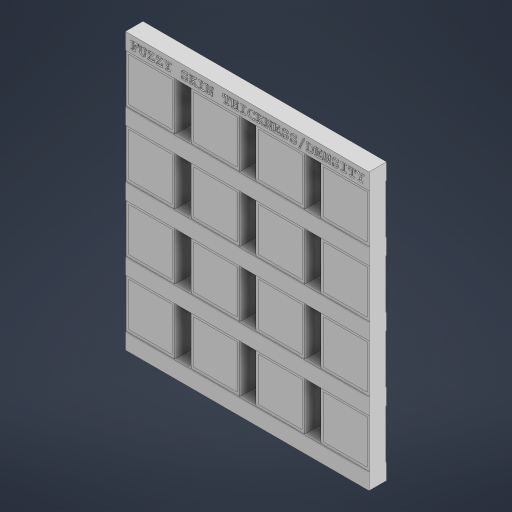
# Autodesk Inventor part: Fuzzy Skin Swatch Module
Saved by Autodesk Inventor 2023.1 (Build 271208000, 208)
## iProperties
Created: 2022-11-27
Part Number: Fuzzy Skin Swatch Module
Material: Generic
Document SubType Name: Modeling
Designer: aubrey-work
Density: 1 g/cm^3
Appearance: Default
Author: aubrey-work
Autodesk Inventor part; units mm, degrees
(part 1 of 2)
ref_plane "YZ Plane" through (0, 0, 0) normal (1, 0, 0) x (0, 1, 0)
ref_plane "XZ Plane" through (0, 0, 0) normal (0, 1, 0) x (-1, 0, 0)
sketch "Sketch1" plane through (0, 0, 0) normal (0, 1, 0) x (-1, 0, 0)
  line L0 (10, -2.7) -> (-10, -2.7)
  line L1 (-10, -2.7) -> (-10, 2.7)
  line L2 (-10, 2.7) -> (10, 2.7)
  line L3 (10, 2.7) -> (10, -2.7)
  line L4 (10, -2.7) -> (-10, 2.7) construction
  line L5 (-10, -2.7) -> (10, 2.7) construction
  point P0 (0, 0)
  dimension "d0" = 20
  dimension "d1" = 5.4
  constraints: 12 end point, 2 midpoint, 2 parallel, 1 horizontal, 1 perpendicular
  measures "d0" distance of L1.end L2.end
  measures "d1" distance of L0.end L1.end
extrude "Bottom Label" add sketch "Sketch1" along normal blind 5
sketch "Sketch2" plane through (0, 5, 0) normal (0, 1, 0) x (1, 0, 0)
  line L0 (-10, -2.5) -> (5, -2.5)
  line L1 (5, -2.5) -> (5, 2.5)
  line L2 (5, 2.5) -> (-10, 2.5)
  line L3 (-10, 2.5) -> (-10, -2.5)
  line L4 (-10, -2.5) -> (5, 2.5) construction
  line L5 (5, -2.5) -> (-10, 2.5) construction
  line L6 (-10, 2.7) -> (-10, -2.7) projected
  point P0 (-2.5, 0)
  point P1 (-2.5, 0)
  point P2 (-10, 0)
  dimension "d4" = 15
  dimension "d5" = 5
  constraints: 12 end point, 4 midpoint, 2 parallel, 1 coincident, 1 horizontal, 1 perpendicular
  measures "d4" distance of L2.end L1.end
  measures "d5" distance of L1.end L0.end
extrude "Tile" add sketch "Sketch2" along normal blind 15
sketch "Sketch7" plane through (-10, 5, 2.5) normal (0, 0, 1) x (1, 0, 0)
  line L0 (15, 0) -> (0, 0) projected
  line L1 (15, 0) -> (15, 15) projected
  line L2 (0, 15) -> (15, 15) projected
  line L3 (0, 0) -> (0, 15) projected
  line L4 (14.2, 14.2) -> (14.2, 0.8)
  line L5 (14.2, 0.8) -> (0.8, 0.8)
  line L6 (0.8, 0.8) -> (0.8, 14.2)
  line L7 (0.8, 14.2) -> (14.2, 14.2)
  point P0 (10, -5)
  dimension "d28" = 0.8
  constraints: 8 end point, 3 other
  measures "d28" distance between parallel lines of L2 L7
extrude "Cut Tile" cut sketch "Sketch7" against normal blind 4.2 contours L4 L5 L6 L7
extrude "Create Tile Inset" add sketch "Sketch7" against normal blind 4.2 separate body contours L4 L5 L6 L7
pattern_linear "Frame Pattern" count 4 spacing 20 along (1, 0, 0) count 4 spacing 20 along (0, 1, 0) of "Tile", "Bottom Label", "Cut Tile" bodies 1
pattern_linear "Tile Insets Rectangular Pattern" count 4 spacing 20 along (1, 0, 0) count 4 spacing 20 along (0, 1, 0) of "Create Tile Inset" bodies 2
sketch "Sketch5" plane through (0, 0, 0) normal (0, 1, 0) x (-1, 0, 0)
  line L0 (-65, 2.7) -> (-70, 2.7)
  line L1 (-70, 2.7) -> (-70, -2.7)
  line L2 (-70, -2.7) -> (-65, -2.7)
  line L3 (-65, -2.7) -> (-65, 2.7)
  line L4 (-65, 2.7) -> (-70, -2.7) construction
  line L5 (-70, 2.7) -> (-65, -2.7) construction
  line L6 (10, -2.7) -> (10, 2.7) projected
  line L7 (6.3576, 0) -> (13.6424, 0) construction
  line L8 (-65, 0) -> (-70, 0) construction
  point P0 (0, 0)
  point P1 (-67.5, 0)
  point P2 (10, 0)
  dimension "d21" = 5
  dimension "d22" = 5.4
  dimension "d23" = 80
  constraints: 16 end point, 6 midpoint, 2 horizontal, 2 parallel, 1 collinear, 1 perpendicular
  measures "d21" distance of L2.end L1.end
  measures "d22" distance of L1.end L0.end
  measures "d23" distance between parallel lines of L6 L1
extrude "Trim Portruding Labels" cut sketch "Sketch5" along normal through all bodies 1
ref_plane "Work Plane1" through (0, 80, 0) normal (0, -1, 0) x (1, 0, 0)
sketch "Sketch6" plane through (0, 80, 0) normal (0, -1, 0) x (1, 0, 0)
  line L0 (65, -2.7) -> (65, 2.7) projected
  line L1 (-10, 2.7) -> (65, 2.7) projected
  line L2 (-10, -2.7) -> (-10, 2.7) projected
  line L3 (65, -2.7) -> (-10, -2.7) projected
  point P0 (0, 0)
extrude "Top Label" add sketch "Sketch6" against normal blind 5 bodies 1
sketch "Sketch4" plane through (-10, 80, 2.7) normal (0, 0, 1) x (1, 0, 0)
  line L0 (0, 5) -> (75, 5) projected
  line L1 (75, 5) -> (75, 0) projected
  line L2 (75, 0) -> (0, 0) projected
  line L3 (0, 0) -> (0, 5) projected
  line L4 (75, -20) -> (0, -20) projected
  line L5 (0, -20) -> (0, -15) projected
  line L6 (0, -15) -> (75, -15) projected
  line L7 (75, -40) -> (0, -40) projected
  line L8 (0, -40) -> (0, -35) projected
  line L9 (0, -35) -> (75, -35) projected
  line L10 (75, -60) -> (0, -60) projected
  line L11 (0, -60) -> (0, -55) projected
  line L12 (0, -55) -> (75, -55) projected
  line L13 (75, -80) -> (0, -80) projected
  line L14 (0, -80) -> (0, -75) projected
  line L15 (0, -75) -> (75, -75) projected
  line L16 (75, -15) -> (75, -20) projected
  line L17 (75, -35) -> (75, -40) projected
  line L18 (75, -55) -> (75, -60) projected
  line L19 (75, -75) -> (75, -80) projected
  line L20 (2.4665, 2.0577) -> (2.4665, 1.4293)
  line L21 (2.4665, 1.4293) -> (2.9052, 1.4293)
  spline S0 degree 2 poles (2.9052, 1.4293) (3.0665, 1.4293) (3.1993, 1.3107) (3.1993, 1.2134) knots 0 0 0 1 2 2 2
  spline S1 degree 2 poles (3.1993, 1.2134) (3.1993, 1.1162) (3.0665, 1) (2.9052, 1) knots 0 0 0 1 2 2 2
  line L22 (2.9052, 1) -> (1.9708, 1)
  spline S2 degree 2 poles (1.9708, 1) (1.8096, 1) (1.6767, 1.1186) (1.6767, 1.2158) knots 0 0 0 1 2 2 2
  spline S3 degree 2 poles (1.6767, 1.2158) (1.6767, 1.3131) (1.8096, 1.4293) (1.9708, 1.4293) knots 0 0 0 1 2 2 2
  line L23 (1.9708, 1.4293) -> (2.0372, 1.4293)
  line L24 (2.0372, 1.4293) -> (2.0372, 3.1107)
  line L25 (2.0372, 3.1107) -> (1.9708, 3.1107)
  spline S4 degree 2 poles (1.9708, 3.1107) (1.8096, 3.1107) (1.6767, 3.2293) (1.6767, 3.3266) knots 0 0 0 1 2 2 2
  spline S5 degree 2 poles (1.6767, 3.3266) (1.6767, 3.4214) (1.8096, 3.54) (1.9708, 3.54) knots 0 0 0 1 2 2 2
  line L26 (1.9708, 3.54) -> (3.9914, 3.5376)
  line L27 (3.9914, 3.5376) -> (3.9914, 2.8854)
  spline S6 degree 2 poles (3.9914, 2.8854) (3.9914, 2.7242) (3.8729, 2.5914) (3.7756, 2.5914) knots 0 0 0 1 2 2 2
  spline S7 degree 2 poles (3.7756, 2.5914) (3.6784, 2.5914) (3.5622, 2.7242) (3.5622, 2.8854) knots 0 0 0 1 2 2 2
  line L28 (3.5622, 2.8854) -> (3.5622, 3.1107)
  line L29 (3.5622, 3.1107) -> (2.4665, 3.1107)
  line L30 (2.4665, 3.1107) -> (2.4665, 2.487)
  line L31 (2.4665, 2.487) -> (2.8436, 2.487)
  spline S8 degree 2 poles (2.8436, 2.487) (2.8436, 2.6483) (2.8815, 2.691) knots 0 0 0 1 1 1
  spline S9 degree 2 poles (2.8815, 2.691) (2.9622, 2.7811) (3.0594, 2.7811) knots 0 0 0 1 1 1
  spline S10 degree 2 poles (3.0594, 2.7811) (3.1566, 2.7811) (3.2728, 2.6483) (3.2728, 2.487) knots 0 0 0 1 2 2 2
  line L32 (3.2728, 2.487) -> (3.2728, 2.0577)
  spline S11 degree 2 poles (3.2728, 2.0577) (3.2728, 1.8965) (3.1543, 1.7637) (3.057, 1.7637) knots 0 0 0 1 2 2 2
  spline S12 degree 2 poles (3.057, 1.7637) (2.9598, 1.7637) (2.8815, 1.8538) knots 0 0 0 1 1 1
  spline S13 degree 2 poles (2.8815, 1.8538) (2.8436, 1.8965) (2.8436, 2.0577) knots 0 0 0 1 1 1
  line L33 (2.8436, 2.0577) -> (2.4665, 2.0577)
  line L34 (6.3156, 3.1084) -> (6.3156, 1.8917)
  spline S14 degree 2 poles (6.3156, 1.8917) (6.3156, 1.4957) (5.7441, 0.9383) (5.3433, 0.9383) knots 0 0 0 1 2 2 2
  spline S15 degree 2 poles (5.3433, 0.9383) (5.1441, 0.9383) (4.7954, 1.0783) (4.5156, 1.351) (4.3614, 1.6451) (4.3614, 1.8917) knots 0 0 0 1 2 3 4 4 4
  line L35 (4.3614, 1.8917) -> (4.3614, 3.1084)
  spline S16 degree 2 poles (4.3614, 3.1084) (4.2001, 3.1084) (4.0673, 3.2269) (4.0673, 3.3242) knots 0 0 0 1 2 2 2
  spline S17 degree 2 poles (4.0673, 3.3242) (4.0673, 3.4214) (4.2001, 3.5376) (4.3614, 3.5376) knots 0 0 0 1 2 2 2
  line L36 (4.3614, 3.5376) -> (4.9448, 3.54)
  spline S18 degree 2 poles (4.9448, 3.54) (5.0848, 3.54) (5.2176, 3.4214) (5.2176, 3.3266) knots 0 0 0 1 2 2 2
  spline S19 degree 2 poles (5.2176, 3.3266) (5.2176, 3.2293) (5.0848, 3.1107) (4.9448, 3.1107) knots 0 0 0 1 2 2 2
  line L37 (4.9448, 3.1107) -> (4.7907, 3.1107)
  line L38 (4.7907, 3.1107) -> (4.7907, 1.8562)
  spline S20 degree 2 poles (4.7907, 1.8562) (4.7907, 1.6641) (5.1108, 1.3676) (5.3362, 1.3676) knots 0 0 0 1 2 2 2
  spline S21 degree 2 poles (5.3362, 1.3676) (5.4879, 1.3676) (5.7512, 1.5099) (5.8342, 1.6475) knots 0 0 0 1 2 2 2
  spline S22 degree 2 poles (5.8342, 1.6475) (5.8864, 1.7328) (5.8864, 1.8562) knots 0 0 0 1 1 1
  line L39 (5.8864, 1.8562) -> (5.8864, 3.1107)
  line L40 (5.8864, 3.1107) -> (5.7322, 3.1107)
  spline S23 degree 2 poles (5.7322, 3.1107) (5.5923, 3.1107) (5.4595, 3.2293) (5.4595, 3.3266) knots 0 0 0 1 2 2 2
  spline S24 degree 2 poles (5.4595, 3.3266) (5.4595, 3.4214) (5.5923, 3.54) (5.7322, 3.54) knots 0 0 0 1 2 2 2
  line L41 (5.7322, 3.54) -> (6.3156, 3.5376)
  spline S25 degree 2 poles (6.3156, 3.5376) (6.4769, 3.5376) (6.6097, 3.4214) (6.6097, 3.3242) knots 0 0 0 1 2 2 2
  spline S26 degree 2 poles (6.6097, 3.3242) (6.6097, 3.2269) (6.4769, 3.1084) (6.3156, 3.1084) knots 0 0 0 1 2 2 2
  line L42 (7.4848, 1.4293) -> (8.4596, 1.4293)
  line L43 (8.4596, 1.4293) -> (8.4596, 1.7471)
  spline S27 degree 2 poles (8.4596, 1.7471) (8.4596, 1.9083) (8.5782, 2.0411) (8.6754, 2.0411) knots 0 0 0 1 2 2 2
  spline S28 degree 2 poles (8.6754, 2.0411) (8.7703, 2.0411) (8.8888, 1.9083) (8.8888, 1.7471) knots 0 0 0 1 2 2 2
  line L44 (8.8888, 1.7471) -> (8.8865, 1)
  line L45 (8.8865, 1) -> (6.937, 1)
  line L46 (6.937, 1) -> (6.937, 1.4293)
  line L47 (6.937, 1.4293) -> (8.2438, 3.1107)
  line L48 (8.2438, 3.1107) -> (7.4564, 3.1107)
  line L49 (7.4564, 3.1107) -> (7.4564, 2.8024)
  spline S29 degree 2 poles (7.4564, 2.8024) (7.4564, 2.6412) (7.3402, 2.5083) (7.2429, 2.5083) knots 0 0 0 1 2 2 2
  spline S30 degree 2 poles (7.2429, 2.5083) (7.1457, 2.5083) (7.0271, 2.6412) (7.0271, 2.8024) knots 0 0 0 1 2 2 2
  line L50 (7.0271, 2.8024) -> (7.0271, 3.54)
  line L51 (7.0271, 3.54) -> (8.7987, 3.5376)
  line L52 (8.7987, 3.5376) -> (8.7987, 3.1202)
  line L53 (8.7987, 3.1202) -> (7.4848, 1.4293)
  line L54 (10.058, 1.4293) -> (11.0328, 1.4293)
  line L55 (11.0328, 1.4293) -> (11.0328, 1.7471)
  spline S31 degree 2 poles (11.0328, 1.7471) (11.0328, 1.9083) (11.1514, 2.0411) (11.2486, 2.0411) knots 0 0 0 1 2 2 2
  spline S32 degree 2 poles (11.2486, 2.0411) (11.3435, 2.0411) (11.462, 1.9083) (11.462, 1.7471) knots 0 0 0 1 2 2 2
  line L56 (11.462, 1.7471) -> (11.4597, 1)
  line L57 (11.4597, 1) -> (9.5102, 1)
  line L58 (9.5102, 1) -> (9.5102, 1.4293)
  line L59 (9.5102, 1.4293) -> (10.817, 3.1107)
  line L60 (10.817, 3.1107) -> (10.0296, 3.1107)
  line L61 (10.0296, 3.1107) -> (10.0296, 2.8024)
  spline S33 degree 2 poles (10.0296, 2.8024) (10.0296, 2.6412) (9.9134, 2.5083) (9.8161, 2.5083) knots 0 0 0 1 2 2 2
  spline S34 degree 2 poles (9.8161, 2.5083) (9.7189, 2.5083) (9.6003, 2.6412) (9.6003, 2.8024) knots 0 0 0 1 2 2 2
  line L62 (9.6003, 2.8024) -> (9.6003, 3.54)
  line L63 (9.6003, 3.54) -> (11.3719, 3.5376)
  line L64 (11.3719, 3.5376) -> (11.3719, 3.1202)
  line L65 (11.3719, 3.1202) -> (10.058, 1.4293)
  line L66 (13.2716, 2.0649) -> (13.2716, 1.4293)
  line L67 (13.2716, 1.4293) -> (13.5609, 1.4293)
  spline S35 degree 2 poles (13.5609, 1.4293) (13.7222, 1.4293) (13.855, 1.3107) (13.855, 1.2134) knots 0 0 0 1 2 2 2
  spline S36 degree 2 poles (13.855, 1.2134) (13.855, 1.1162) (13.7222, 1) (13.5609, 1) knots 0 0 0 1 2 2 2
  line L68 (13.5609, 1) -> (12.553, 1)
  spline S37 degree 2 poles (12.553, 1) (12.3917, 1) (12.2589, 1.1186) (12.2589, 1.2158) knots 0 0 0 1 2 2 2
  spline S38 degree 2 poles (12.2589, 1.2158) (12.2589, 1.3131) (12.3917, 1.4293) (12.553, 1.4293) knots 0 0 0 1 2 2 2
  line L69 (12.553, 1.4293) -> (12.8423, 1.4293)
  line L70 (12.8423, 1.4293) -> (12.8423, 2.0649)
  line L71 (12.8423, 2.0649) -> (12.1308, 3.1131)
  spline S39 degree 2 poles (12.1308, 3.1131) (11.9696, 3.1131) (11.8368, 3.2317) (11.8368, 3.3289) knots 0 0 0 1 2 2 2
  spline S40 degree 2 poles (11.8368, 3.3289) (11.8368, 3.4238) (11.9696, 3.5424) (12.1308, 3.5424) knots 0 0 0 1 2 2 2
  line L72 (12.1308, 3.5424) -> (12.534, 3.54)
  spline S41 degree 2 poles (12.534, 3.54) (12.6905, 3.54) (12.8233, 3.4238) (12.8233, 3.3266) knots 0 0 0 1 2 2 2
  spline S42 degree 2 poles (12.8233, 3.3266) (12.8233, 3.1819) (12.6502, 3.1107) knots 0 0 0 1 1 1
  line L73 (12.6502, 3.1107) -> (13.0581, 2.5107)
  line L74 (13.0581, 2.5107) -> (13.4637, 3.1107)
  spline S43 degree 2 poles (13.4637, 3.1107) (13.3024, 3.1107) (13.1696, 3.2293) (13.1696, 3.3266) knots 0 0 0 1 2 2 2
  spline S44 degree 2 poles (13.1696, 3.3266) (13.1696, 3.4214) (13.3024, 3.54) (13.4637, 3.54) knots 0 0 0 1 2 2 2
  line L75 (13.4637, 3.54) -> (13.9807, 3.54)
  spline S45 degree 2 poles (13.9807, 3.54) (14.1396, 3.54) (14.2724, 3.4238) (14.2724, 3.3266) knots 0 0 0 1 2 2 2
  spline S46 degree 2 poles (14.2724, 3.3266) (14.2724, 3.2293) (14.1396, 3.1107) (13.9807, 3.1107) knots 0 0 0 1 2 2 2
  line L76 (13.9807, 3.1107) -> (13.2716, 2.0649)
  spline S47 degree 2 poles (17.5737, 1.1091) (17.5168, 1.0427) (17.448, 1.0047) (17.3982, 1.0047) knots 0 0 0 1 2 2 2
  spline S48 degree 2 poles (17.3982, 1.0047) (17.2986, 1.0047) (17.18, 1.1376) (17.18, 1.2893) knots 0 0 0 1 2 2 2
  line L77 (17.18, 1.2893) -> (17.18, 1.5787)
  spline S49 degree 2 poles (17.18, 1.5787) (17.18, 1.7328) (17.2986, 1.8656) (17.3982, 1.8656) knots 0 0 0 1 2 2 2
  spline S50 degree 2 poles (17.3982, 1.8656) (17.4741, 1.8656) (17.5761, 1.785) (17.6306, 1.6) (17.6591, 1.5668) knots 0 0 0 1 2 3 3 3
  spline S51 degree 2 poles (17.6591, 1.5668) (17.7207, 1.5004) (18.029, 1.3676) (18.2117, 1.3676) knots 0 0 0 1 2 2 2
  spline S52 degree 2 poles (18.2117, 1.3676) (18.4986, 1.3676) (18.6836, 1.5004) knots 0 0 0 1 1 1
  spline S53 degree 2 poles (18.6836, 1.5004) (18.7998, 1.5834) (18.7998, 1.702) knots 0 0 0 1 1 1
  spline S54 degree 2 poles (18.7998, 1.702) (18.7998, 1.7826) (18.6883, 1.9226) (18.5603, 1.9676) knots 0 0 0 1 2 2 2
  spline S55 degree 2 poles (18.5603, 1.9676) (18.4773, 1.9985) (18.1879, 2.053) knots 0 0 0 1 1 1
  spline S56 degree 2 poles (18.1879, 2.053) (17.8369, 2.1194) (17.4765, 2.302) (17.2654, 2.6364) (17.2654, 2.8309) knots 0 0 0 1 2 3 3 3
  spline S57 degree 2 poles (17.2654, 2.8309) (17.2654, 3.1392) (17.78, 3.6017) (18.1927, 3.6017) knots 0 0 0 1 2 2 2
  spline S58 degree 2 poles (18.1927, 3.6017) (18.3587, 3.6017) (18.6409, 3.5281) (18.7571, 3.4523) knots 0 0 0 1 2 2 2
  spline S59 degree 2 poles (18.7571, 3.4523) (18.8401, 3.5353) (18.9255, 3.5353) knots 0 0 0 1 1 1
  spline S60 degree 2 poles (18.9255, 3.5353) (19.0204, 3.5353) (19.139, 3.4024) (19.139, 3.2507) knots 0 0 0 1 2 2 2
  line L78 (19.139, 3.2507) -> (19.139, 2.9281)
  spline S61 degree 2 poles (19.139, 2.9281) (19.139, 2.774) (19.0204, 2.6412) (18.9255, 2.6412) knots 0 0 0 1 2 2 2
  spline S62 degree 2 poles (18.9255, 2.6412) (18.8472, 2.6412) (18.788, 2.6886) knots 0 0 0 1 1 1
  spline S63 degree 2 poles (18.788, 2.6886) (18.7405, 2.7242) (18.6955, 2.9376) (18.6599, 2.985) knots 0 0 0 1 2 2 2
  spline S64 degree 2 poles (18.6599, 2.985) (18.5982, 3.0633) (18.3563, 3.1724) (18.1974, 3.1724) knots 0 0 0 1 2 2 2
  spline S65 degree 2 poles (18.1974, 3.1724) (17.965, 3.1724) (17.6946, 2.9566) (17.6946, 2.8404) knots 0 0 0 1 2 2 2
  spline S66 degree 2 poles (17.6946, 2.8404) (17.6946, 2.7597) (17.8061, 2.6127) (17.9105, 2.57) knots 0 0 0 1 2 2 2
  spline S67 degree 2 poles (17.9105, 2.57) (17.9816, 2.5416) (18.6385, 2.4111) (18.9943, 2.257) (19.2291, 1.9249) (19.2291, 1.6973) knots 0 0 0 1 2 3 4 4 4
  spline S68 degree 2 poles (19.2291, 1.6973) (19.2291, 1.3795) (19.0061, 1.1897) knots 0 0 0 1 1 1
  spline S69 degree 2 poles (19.0061, 1.1897) (18.7073, 0.9383) (18.2472, 0.9383) knots 0 0 0 1 1 1
  spline S70 degree 2 poles (18.2472, 0.9383) (18.0694, 0.9383) (17.7326, 1.0237) (17.5737, 1.1091) knots 0 0 0 1 2 2 2
  line L79 (20.3271, 1.9083) -> (20.3271, 1.4293)
  line L80 (20.3271, 1.4293) -> (20.4813, 1.4293)
  spline S71 degree 2 poles (20.4813, 1.4293) (20.6212, 1.4293) (20.754, 1.3107) (20.754, 1.2134) knots 0 0 0 1 2 2 2
  spline S72 degree 2 poles (20.754, 1.2134) (20.754, 1.1162) (20.6212, 1) (20.4813, 1) knots 0 0 0 1 2 2 2
  line L81 (20.4813, 1) -> (19.8315, 1)
  spline S73 degree 2 poles (19.8315, 1) (19.6915, 1) (19.5587, 1.1186) (19.5587, 1.2158) knots 0 0 0 1 2 2 2
  spline S74 degree 2 poles (19.5587, 1.2158) (19.5587, 1.3131) (19.6915, 1.4293) (19.8315, 1.4293) knots 0 0 0 1 2 2 2
  line L82 (19.8315, 1.4293) -> (19.8979, 1.4293)
  line L83 (19.8979, 1.4293) -> (19.8979, 3.1107)
  line L84 (19.8979, 3.1107) -> (19.8315, 3.1107)
  spline S75 degree 2 poles (19.8315, 3.1107) (19.6915, 3.1107) (19.5587, 3.2293) (19.5587, 3.3266) knots 0 0 0 1 2 2 2
  spline S76 degree 2 poles (19.5587, 3.3266) (19.5587, 3.4214) (19.6915, 3.54) (19.8315, 3.54) knots 0 0 0 1 2 2 2
  line L85 (19.8315, 3.54) -> (20.4813, 3.5376)
  spline S77 degree 2 poles (20.4813, 3.5376) (20.6212, 3.5376) (20.754, 3.4214) (20.754, 3.3242) knots 0 0 0 1 2 2 2
  spline S78 degree 2 poles (20.754, 3.3242) (20.754, 3.2269) (20.6212, 3.1084) (20.4813, 3.1084) knots 0 0 0 1 2 2 2
  line L86 (20.4813, 3.1084) -> (20.3271, 3.1084)
  line L87 (20.3271, 3.1084) -> (20.3271, 2.4728)
  line L88 (20.3271, 2.4728) -> (21.0884, 3.1273)
  spline S79 degree 2 poles (21.0884, 3.1273) (21.1027, 3.1273) (20.9698, 3.2246) (20.9698, 3.3218) knots 0 0 0 1 2 2 2
  spline S80 degree 2 poles (20.9698, 3.3218) (20.9698, 3.4167) (21.1027, 3.54) (21.0884, 3.54) knots 0 0 0 1 2 2 2
  line L89 (21.0884, 3.54) -> (21.7098, 3.5376)
  spline S81 degree 2 poles (21.7098, 3.5376) (21.8711, 3.5376) (22.0039, 3.4214) (22.0039, 3.3242) knots 0 0 0 1 2 2 2
  spline S82 degree 2 poles (22.0039, 3.3242) (22.0039, 3.2269) (21.8711, 3.1084) (21.7098, 3.1084) knots 0 0 0 1 2 2 2
  line L90 (21.7098, 3.1084) -> (20.939, 2.4396)
  spline S83 degree 2 poles (20.939, 2.4396) (21.1548, 2.3139) (21.5343, 1.8063) (21.6813, 1.4293) knots 0 0 0 1 2 2 2
  line L91 (21.6813, 1.4293) -> (21.7975, 1.4293)
  spline S84 degree 2 poles (21.7975, 1.4293) (21.9588, 1.4293) (22.0916, 1.3107) (22.0916, 1.2134) knots 0 0 0 1 2 2 2
  spline S85 degree 2 poles (22.0916, 1.2134) (22.0916, 1.1162) (21.9588, 1) (21.7975, 1) knots 0 0 0 1 2 2 2
  line L92 (21.7975, 1) -> (21.4062, 1)
  spline S86 degree 2 poles (21.4062, 1) (21.2734, 1.3225) (21.1145, 1.6142) knots 0 0 0 1 1 1
  spline S87 degree 2 poles (21.1145, 1.6142) (20.9841, 1.8514) (20.7517, 2.0672) (20.5904, 2.1336) knots 0 0 0 1 2 2 2
  line L93 (20.5904, 2.1336) -> (20.3271, 1.9083)
  line L94 (23.562, 3.1084) -> (23.562, 1.4293)
  line L95 (23.562, 1.4293) -> (23.996, 1.4293)
  spline S88 degree 2 poles (23.996, 1.4293) (24.1573, 1.4293) (24.2901, 1.3107) (24.2901, 1.2134) knots 0 0 0 1 2 2 2
  spline S89 degree 2 poles (24.2901, 1.2134) (24.2901, 1.1162) (24.1573, 1) (23.996, 1) knots 0 0 0 1 2 2 2
  line L96 (23.996, 1) -> (22.6987, 1)
  spline S90 degree 2 poles (22.6987, 1) (22.5375, 1) (22.4047, 1.1186) (22.4047, 1.2158) knots 0 0 0 1 2 2 2
  spline S91 degree 2 poles (22.4047, 1.2158) (22.4047, 1.3131) (22.5375, 1.4293) (22.6987, 1.4293) knots 0 0 0 1 2 2 2
  line L97 (22.6987, 1.4293) -> (23.1328, 1.4293)
  line L98 (23.1328, 1.4293) -> (23.1328, 3.1107)
  line L99 (23.1328, 3.1107) -> (22.6987, 3.1107)
  spline S92 degree 2 poles (22.6987, 3.1107) (22.5375, 3.1107) (22.4047, 3.2293) (22.4047, 3.3266) knots 0 0 0 1 2 2 2
  spline S93 degree 2 poles (22.4047, 3.3266) (22.4047, 3.4214) (22.5375, 3.54) (22.6987, 3.54) knots 0 0 0 1 2 2 2
  line L100 (22.6987, 3.54) -> (23.996, 3.5376)
  spline S94 degree 2 poles (23.996, 3.5376) (24.1573, 3.5376) (24.2901, 3.4214) (24.2901, 3.3242) knots 0 0 0 1 2 2 2
  spline S95 degree 2 poles (24.2901, 3.3242) (24.2901, 3.2269) (24.1573, 3.1084) (23.996, 3.1084) knots 0 0 0 1 2 2 2
  line L101 (23.996, 3.1084) -> (23.562, 3.1084)
  line L102 (25.3834, 2.7265) -> (25.3834, 1.4293)
  line L103 (25.3834, 1.4293) -> (25.5376, 1.4293)
  spline S96 degree 2 poles (25.5376, 1.4293) (25.6988, 1.4293) (25.8317, 1.3107) (25.8317, 1.2134) knots 0 0 0 1 2 2 2
  spline S97 degree 2 poles (25.8317, 1.2134) (25.8317, 1.1162) (25.6988, 1) (25.5376, 1) knots 0 0 0 1 2 2 2
  line L104 (25.5376, 1) -> (24.9542, 1)
  spline S98 degree 2 poles (24.9542, 1) (24.7929, 1) (24.6601, 1.1186) (24.6601, 1.2158) knots 0 0 0 1 2 2 2
  spline S99 degree 2 poles (24.6601, 1.2158) (24.6601, 1.3131) (24.7929, 1.4293) (24.9542, 1.4293) knots 0 0 0 1 2 2 2
  line L105 (24.9542, 1.4293) -> (24.9542, 3.1107)
  line L106 (24.9542, 3.1107) -> (24.8878, 3.1107)
  spline S100 degree 2 poles (24.8878, 3.1107) (24.7265, 3.1107) (24.5937, 3.2293) (24.5937, 3.3266) knots 0 0 0 1 2 2 2
  spline S101 degree 2 poles (24.5937, 3.3266) (24.5937, 3.4214) (24.7265, 3.54) (24.8878, 3.54) knots 0 0 0 1 2 2 2
  line L107 (24.8878, 3.54) -> (25.381, 3.5376)
  line L108 (25.381, 3.5376) -> (26.4838, 1.8158)
  line L109 (26.4838, 1.8158) -> (26.4838, 3.1107)
  line L110 (26.4838, 3.1107) -> (26.3297, 3.1107)
  spline S102 degree 2 poles (26.3297, 3.1107) (26.1684, 3.1107) (26.0356, 3.2293) (26.0356, 3.3266) knots 0 0 0 1 2 2 2
  spline S103 degree 2 poles (26.0356, 3.3266) (26.0356, 3.4214) (26.1684, 3.54) (26.3297, 3.54) knots 0 0 0 1 2 2 2
  line L111 (26.3297, 3.54) -> (26.9131, 3.5376)
  spline S104 degree 2 poles (26.9131, 3.5376) (27.0744, 3.5376) (27.2072, 3.4214) (27.2072, 3.3242) knots 0 0 0 1 2 2 2
  spline S105 degree 2 poles (27.2072, 3.3242) (27.2072, 3.2269) (27.0744, 3.1084) (26.9131, 3.1084) knots 0 0 0 1 2 2 2
  line L112 (26.9131, 3.1084) -> (26.9131, 1)
  line L113 (26.9131, 1) -> (26.491, 1)
  line L114 (26.491, 1) -> (25.3834, 2.7265)
  line L115 (31.3148, 3.1107) -> (31.3148, 1.4293)
  line L116 (31.3148, 1.4293) -> (31.6042, 1.4293)
  spline S106 degree 2 poles (31.6042, 1.4293) (31.7654, 1.4293) (31.8982, 1.3107) (31.8982, 1.2134) knots 0 0 0 1 2 2 2
  spline S107 degree 2 poles (31.8982, 1.2134) (31.8982, 1.1162) (31.7654, 1) (31.6042, 1) knots 0 0 0 1 2 2 2
  line L117 (31.6042, 1) -> (30.5986, 1)
  spline S108 degree 2 poles (30.5986, 1) (30.4373, 1) (30.3045, 1.1186) (30.3045, 1.2158) knots 0 0 0 1 2 2 2
  spline S109 degree 2 poles (30.3045, 1.2158) (30.3045, 1.3131) (30.4373, 1.4293) (30.5986, 1.4293) knots 0 0 0 1 2 2 2
  line L118 (30.5986, 1.4293) -> (30.8856, 1.4293)
  line L119 (30.8856, 1.4293) -> (30.8856, 3.1107)
  line L120 (30.8856, 3.1107) -> (30.4207, 3.1107)
  line L121 (30.4207, 3.1107) -> (30.4207, 2.7052)
  spline S110 degree 2 poles (30.4207, 2.7052) (30.4207, 2.5439) (30.3021, 2.4111) (30.2049, 2.4111) knots 0 0 0 1 2 2 2
  spline S111 degree 2 poles (30.2049, 2.4111) (30.1077, 2.4111) (29.9915, 2.5439) (29.9915, 2.7052) knots 0 0 0 1 2 2 2
  line L122 (29.9915, 2.7052) -> (29.9915, 3.54)
  line L123 (29.9915, 3.54) -> (32.216, 3.54)
  line L124 (32.216, 3.54) -> (32.216, 2.7052)
  spline S112 degree 2 poles (32.216, 2.7052) (32.216, 2.5439) (32.0975, 2.4111) (32.0002, 2.4111) knots 0 0 0 1 2 2 2
  spline S113 degree 2 poles (32.0002, 2.4111) (31.903, 2.4111) (31.7868, 2.5439) (31.7868, 2.7052) knots 0 0 0 1 2 2 2
  line L125 (31.7868, 2.7052) -> (31.7868, 3.1107)
  line L126 (31.7868, 3.1107) -> (31.3148, 3.1107)
  line L127 (34.1513, 2.0506) -> (33.2335, 2.0506)
  line L128 (33.2335, 2.0506) -> (33.2335, 1.4293)
  line L129 (33.2335, 1.4293) -> (33.2999, 1.4293)
  spline S114 degree 2 poles (33.2999, 1.4293) (33.4398, 1.4293) (33.5726, 1.3107) (33.5726, 1.2134) knots 0 0 0 1 2 2 2
  spline S115 degree 2 poles (33.5726, 1.2134) (33.5726, 1.1162) (33.4398, 1) (33.2999, 1) knots 0 0 0 1 2 2 2
  line L130 (33.2999, 1) -> (32.8042, 1)
  spline S116 degree 2 poles (32.8042, 1) (32.6643, 1) (32.5315, 1.1186) (32.5315, 1.2158) knots 0 0 0 1 2 2 2
  spline S117 degree 2 poles (32.5315, 1.2158) (32.5315, 1.3131) (32.6192, 1.3889) knots 0 0 0 1 1 1
  spline S118 degree 2 poles (32.6192, 1.3889) (32.6643, 1.4293) (32.8042, 1.4293) knots 0 0 0 1 1 1
  line L131 (32.8042, 1.4293) -> (32.8042, 3.1107)
  spline S119 degree 2 poles (32.8042, 3.1107) (32.6643, 3.1107) (32.5315, 3.2293) (32.5315, 3.3266) knots 0 0 0 1 2 2 2
  spline S120 degree 2 poles (32.5315, 3.3266) (32.5315, 3.4214) (32.6643, 3.54) (32.8042, 3.54) knots 0 0 0 1 2 2 2
  line L132 (32.8042, 3.54) -> (33.2999, 3.5376)
  spline S121 degree 2 poles (33.2999, 3.5376) (33.4398, 3.5376) (33.5726, 3.4214) (33.5726, 3.3242) knots 0 0 0 1 2 2 2
  spline S122 degree 2 poles (33.5726, 3.3242) (33.5726, 3.2269) (33.4398, 3.1084) (33.2999, 3.1084) knots 0 0 0 1 2 2 2
  line L133 (33.2999, 3.1084) -> (33.2335, 3.1084)
  line L134 (33.2335, 3.1084) -> (33.2335, 2.4799)
  line L135 (33.2335, 2.4799) -> (34.1513, 2.4799)
  line L136 (34.1513, 2.4799) -> (34.1513, 3.1107)
  line L137 (34.1513, 3.1107) -> (34.0849, 3.1107)
  spline S123 degree 2 poles (34.0849, 3.1107) (33.945, 3.1107) (33.8121, 3.2293) (33.8121, 3.3266) knots 0 0 0 1 2 2 2
  spline S124 degree 2 poles (33.8121, 3.3266) (33.8121, 3.4214) (33.945, 3.54) (34.0849, 3.54) knots 0 0 0 1 2 2 2
  line L138 (34.0849, 3.54) -> (34.5805, 3.5376)
  spline S125 degree 2 poles (34.5805, 3.5376) (34.7205, 3.5376) (34.8533, 3.4214) (34.8533, 3.3242) knots 0 0 0 1 2 2 2
  spline S126 degree 2 poles (34.8533, 3.3242) (34.8533, 3.2269) (34.7205, 3.1084) (34.5805, 3.1084) knots 0 0 0 1 2 2 2
  line L139 (34.5805, 3.1084) -> (34.5805, 1.4293)
  spline S127 degree 2 poles (34.5805, 1.4293) (34.7205, 1.4293) (34.7632, 1.3913) knots 0 0 0 1 1 1
  spline S128 degree 2 poles (34.7632, 1.3913) (34.8533, 1.3107) (34.8533, 1.2134) knots 0 0 0 1 1 1
  spline S129 degree 2 poles (34.8533, 1.2134) (34.8533, 1.1162) (34.7205, 1) (34.5805, 1) knots 0 0 0 1 2 2 2
  line L140 (34.5805, 1) -> (34.0849, 1)
  spline S130 degree 2 poles (34.0849, 1) (33.945, 1) (33.8121, 1.1186) (33.8121, 1.2158) knots 0 0 0 1 2 2 2
  spline S131 degree 2 poles (33.8121, 1.2158) (33.8121, 1.3131) (33.945, 1.4293) (34.0849, 1.4293) knots 0 0 0 1 2 2 2
  line L141 (34.0849, 1.4293) -> (34.1513, 1.4293)
  line L142 (34.1513, 1.4293) -> (34.1513, 2.0506)
  line L143 (36.4683, 3.1084) -> (36.4683, 1.4293)
  line L144 (36.4683, 1.4293) -> (36.9024, 1.4293)
  spline S132 degree 2 poles (36.9024, 1.4293) (37.0636, 1.4293) (37.1964, 1.3107) (37.1964, 1.2134) knots 0 0 0 1 2 2 2
  spline S133 degree 2 poles (37.1964, 1.2134) (37.1964, 1.1162) (37.0636, 1) (36.9024, 1) knots 0 0 0 1 2 2 2
  line L145 (36.9024, 1) -> (35.6051, 1)
  spline S134 degree 2 poles (35.6051, 1) (35.4438, 1) (35.311, 1.1186) (35.311, 1.2158) knots 0 0 0 1 2 2 2
  spline S135 degree 2 poles (35.311, 1.2158) (35.311, 1.3131) (35.4438, 1.4293) (35.6051, 1.4293) knots 0 0 0 1 2 2 2
  line L146 (35.6051, 1.4293) -> (36.0391, 1.4293)
  line L147 (36.0391, 1.4293) -> (36.0391, 3.1107)
  line L148 (36.0391, 3.1107) -> (35.6051, 3.1107)
  spline S136 degree 2 poles (35.6051, 3.1107) (35.4438, 3.1107) (35.311, 3.2293) (35.311, 3.3266) knots 0 0 0 1 2 2 2
  spline S137 degree 2 poles (35.311, 3.3266) (35.311, 3.4214) (35.4438, 3.54) (35.6051, 3.54) knots 0 0 0 1 2 2 2
  line L149 (35.6051, 3.54) -> (36.9024, 3.5376)
  spline S138 degree 2 poles (36.9024, 3.5376) (37.0636, 3.5376) (37.1964, 3.4214) (37.1964, 3.3242) knots 0 0 0 1 2 2 2
  spline S139 degree 2 poles (37.1964, 3.3242) (37.1964, 3.2269) (37.0636, 3.1084) (36.9024, 3.1084) knots 0 0 0 1 2 2 2
  line L150 (36.9024, 3.1084) -> (36.4683, 3.1084)
  spline S140 degree 2 poles (39.4993, 3.4285) (39.5396, 3.4831) (39.6345, 3.5376) (39.689, 3.5376) knots 0 0 0 1 2 2 2
  spline S141 degree 2 poles (39.689, 3.5376) (39.7839, 3.5376) (39.9024, 3.4072) (39.9024, 3.253) knots 0 0 0 1 2 2 2
  line L151 (39.9024, 3.253) -> (39.9024, 2.8878)
  spline S142 degree 2 poles (39.9024, 2.8878) (39.9024, 2.7337) (39.7839, 2.6008) (39.689, 2.6008) knots 0 0 0 1 2 2 2
  spline S143 degree 2 poles (39.689, 2.6008) (39.6036, 2.6008) (39.5514, 2.6483) knots 0 0 0 1 1 1
  spline S144 degree 2 poles (39.5514, 2.6483) (39.4993, 2.6981) (39.4732, 2.8285) knots 0 0 0 1 1 1
  spline S145 degree 2 poles (39.4732, 2.8285) (39.459, 2.9163) (39.4139, 2.9661) knots 0 0 0 1 1 1
  spline S146 degree 2 poles (39.4139, 2.9661) (39.3285, 3.0586) (39.0202, 3.1724) (38.8661, 3.1724) knots 0 0 0 1 2 2 2
  spline S147 degree 2 poles (38.8661, 3.1724) (38.674, 3.1724) (38.3514, 3.004) (38.1048, 2.6293) (38.1048, 2.3684) knots 0 0 0 1 2 3 3 3
  line L152 (38.1048, 2.3684) -> (38.1048, 2.0909)
  spline S148 degree 2 poles (38.1048, 2.0909) (38.1048, 1.7826) (38.5554, 1.3676) (38.9538, 1.3676) knots 0 0 0 1 2 2 2
  spline S149 degree 2 poles (38.9538, 1.3676) (39.1933, 1.3676) (39.357, 1.4316) knots 0 0 0 1 1 1
  spline S150 degree 2 poles (39.357, 1.4316) (39.4542, 1.4696) (39.5633, 1.581) knots 0 0 0 1 1 1
  spline S151 degree 2 poles (39.5633, 1.581) (39.6297, 1.6475) (39.7056, 1.6878) (39.753, 1.6878) knots 0 0 0 1 2 2 2
  spline S152 degree 2 poles (39.753, 1.6878) (39.8384, 1.6878) (39.9689, 1.5573) (39.9689, 1.4696) knots 0 0 0 1 2 2 2
  spline S153 degree 2 poles (39.9689, 1.4696) (39.9689, 1.3818) (39.8811, 1.2822) knots 0 0 0 1 1 1
  spline S154 degree 2 poles (39.8811, 1.2822) (39.753, 1.1352) (39.5514, 1.0522) knots 0 0 0 1 1 1
  spline S155 degree 2 poles (39.5514, 1.0522) (39.2835, 0.9383) (38.9562, 0.9383) knots 0 0 0 1 1 1
  spline S156 degree 2 poles (38.9562, 0.9383) (38.5743, 0.9383) (38.2708, 1.0949) knots 0 0 0 1 1 1
  spline S157 degree 2 poles (38.2708, 1.0949) (38.0218, 1.2206) (37.6755, 1.7637) (37.6755, 2.0838) knots 0 0 0 1 2 2 2
  line L153 (37.6755, 2.0838) -> (37.6755, 2.3732)
  spline S158 degree 2 poles (37.6755, 2.3732) (37.6755, 2.7076) (37.9862, 3.2886) (38.5388, 3.6017) (38.8495, 3.6017) knots 0 0 0 1 2 3 3 3
  spline S159 degree 2 poles (38.8495, 3.6017) (39.0344, 3.6017) (39.3593, 3.5163) (39.4993, 3.4285) knots 0 0 0 1 2 2 2
  line L154 (40.9531, 1.9083) -> (40.9531, 1.4293)
  line L155 (40.9531, 1.4293) -> (41.1072, 1.4293)
  spline S160 degree 2 poles (41.1072, 1.4293) (41.2472, 1.4293) (41.38, 1.3107) (41.38, 1.2134) knots 0 0 0 1 2 2 2
  spline S161 degree 2 poles (41.38, 1.2134) (41.38, 1.1162) (41.2472, 1) (41.1072, 1) knots 0 0 0 1 2 2 2
  line L156 (41.1072, 1) -> (40.4574, 1)
  spline S162 degree 2 poles (40.4574, 1) (40.3175, 1) (40.1847, 1.1186) (40.1847, 1.2158) knots 0 0 0 1 2 2 2
  spline S163 degree 2 poles (40.1847, 1.2158) (40.1847, 1.3131) (40.3175, 1.4293) (40.4574, 1.4293) knots 0 0 0 1 2 2 2
  line L157 (40.4574, 1.4293) -> (40.5238, 1.4293)
  line L158 (40.5238, 1.4293) -> (40.5238, 3.1107)
  line L159 (40.5238, 3.1107) -> (40.4574, 3.1107)
  spline S164 degree 2 poles (40.4574, 3.1107) (40.3175, 3.1107) (40.1847, 3.2293) (40.1847, 3.3266) knots 0 0 0 1 2 2 2
  spline S165 degree 2 poles (40.1847, 3.3266) (40.1847, 3.4214) (40.3175, 3.54) (40.4574, 3.54) knots 0 0 0 1 2 2 2
  line L160 (40.4574, 3.54) -> (41.1072, 3.5376)
  spline S166 degree 2 poles (41.1072, 3.5376) (41.2472, 3.5376) (41.38, 3.4214) (41.38, 3.3242) knots 0 0 0 1 2 2 2
  spline S167 degree 2 poles (41.38, 3.3242) (41.38, 3.2269) (41.2472, 3.1084) (41.1072, 3.1084) knots 0 0 0 1 2 2 2
  line L161 (41.1072, 3.1084) -> (40.9531, 3.1084)
  line L162 (40.9531, 3.1084) -> (40.9531, 2.4728)
  line L163 (40.9531, 2.4728) -> (41.7144, 3.1273)
  spline S168 degree 2 poles (41.7144, 3.1273) (41.7286, 3.1273) (41.5958, 3.2246) (41.5958, 3.3218) knots 0 0 0 1 2 2 2
  spline S169 degree 2 poles (41.5958, 3.3218) (41.5958, 3.4167) (41.7286, 3.54) (41.7144, 3.54) knots 0 0 0 1 2 2 2
  line L164 (41.7144, 3.54) -> (42.3357, 3.5376)
  spline S170 degree 2 poles (42.3357, 3.5376) (42.497, 3.5376) (42.6298, 3.4214) (42.6298, 3.3242) knots 0 0 0 1 2 2 2
  spline S171 degree 2 poles (42.6298, 3.3242) (42.6298, 3.2269) (42.497, 3.1084) (42.3357, 3.1084) knots 0 0 0 1 2 2 2
  line L165 (42.3357, 3.1084) -> (41.565, 2.4396)
  spline S172 degree 2 poles (41.565, 2.4396) (41.7808, 2.3139) (42.1602, 1.8063) (42.3073, 1.4293) knots 0 0 0 1 2 2 2
  line L166 (42.3073, 1.4293) -> (42.4235, 1.4293)
  spline S173 degree 2 poles (42.4235, 1.4293) (42.5847, 1.4293) (42.7176, 1.3107) (42.7176, 1.2134) knots 0 0 0 1 2 2 2
  spline S174 degree 2 poles (42.7176, 1.2134) (42.7176, 1.1162) (42.5847, 1) (42.4235, 1) knots 0 0 0 1 2 2 2
  line L167 (42.4235, 1) -> (42.0322, 1)
  spline S175 degree 2 poles (42.0322, 1) (41.8993, 1.3225) (41.7405, 1.6142) knots 0 0 0 1 1 1
  spline S176 degree 2 poles (41.7405, 1.6142) (41.61, 1.8514) (41.3776, 2.0672) (41.2163, 2.1336) knots 0 0 0 1 2 2 2
  line L168 (41.2163, 2.1336) -> (40.9531, 1.9083)
  line L169 (43.4362, 2.7265) -> (43.4362, 1.4293)
  line L170 (43.4362, 1.4293) -> (43.5903, 1.4293)
  spline S177 degree 2 poles (43.5903, 1.4293) (43.7516, 1.4293) (43.8844, 1.3107) (43.8844, 1.2134) knots 0 0 0 1 2 2 2
  spline S178 degree 2 poles (43.8844, 1.2134) (43.8844, 1.1162) (43.7516, 1) (43.5903, 1) knots 0 0 0 1 2 2 2
  line L171 (43.5903, 1) -> (43.0069, 1)
  spline S179 degree 2 poles (43.0069, 1) (42.8456, 1) (42.7128, 1.1186) (42.7128, 1.2158) knots 0 0 0 1 2 2 2
  spline S180 degree 2 poles (42.7128, 1.2158) (42.7128, 1.3131) (42.8456, 1.4293) (43.0069, 1.4293) knots 0 0 0 1 2 2 2
  line L172 (43.0069, 1.4293) -> (43.0069, 3.1107)
  line L173 (43.0069, 3.1107) -> (42.9405, 3.1107)
  spline S181 degree 2 poles (42.9405, 3.1107) (42.7792, 3.1107) (42.6464, 3.2293) (42.6464, 3.3266) knots 0 0 0 1 2 2 2
  spline S182 degree 2 poles (42.6464, 3.3266) (42.6464, 3.4214) (42.7792, 3.54) (42.9405, 3.54) knots 0 0 0 1 2 2 2
  line L174 (42.9405, 3.54) -> (43.4338, 3.5376)
  line L175 (43.4338, 3.5376) -> (44.5366, 1.8158)
  line L176 (44.5366, 1.8158) -> (44.5366, 3.1107)
  line L177 (44.5366, 3.1107) -> (44.3824, 3.1107)
  spline S183 degree 2 poles (44.3824, 3.1107) (44.2212, 3.1107) (44.0884, 3.2293) (44.0884, 3.3266) knots 0 0 0 1 2 2 2
  spline S184 degree 2 poles (44.0884, 3.3266) (44.0884, 3.4214) (44.2212, 3.54) (44.3824, 3.54) knots 0 0 0 1 2 2 2
  line L178 (44.3824, 3.54) -> (44.9658, 3.5376)
  spline S185 degree 2 poles (44.9658, 3.5376) (45.1271, 3.5376) (45.2599, 3.4214) (45.2599, 3.3242) knots 0 0 0 1 2 2 2
  spline S186 degree 2 poles (45.2599, 3.3242) (45.2599, 3.2269) (45.1271, 3.1084) (44.9658, 3.1084) knots 0 0 0 1 2 2 2
  line L179 (44.9658, 3.1084) -> (44.9658, 1)
  line L180 (44.9658, 1) -> (44.5437, 1)
  line L181 (44.5437, 1) -> (43.4362, 2.7265)
  line L182 (46.1469, 2.0601) -> (46.1469, 1.4293)
  line L183 (46.1469, 1.4293) -> (47.2426, 1.4293)
  line L184 (47.2426, 1.4293) -> (47.2426, 1.6617)
  spline S187 degree 2 poles (47.2426, 1.6617) (47.2426, 1.823) (47.3612, 1.9558) (47.4584, 1.9558) knots 0 0 0 1 2 2 2
  spline S188 degree 2 poles (47.4584, 1.9558) (47.5557, 1.9558) (47.6719, 1.823) (47.6719, 1.6617) knots 0 0 0 1 2 2 2
  line L185 (47.6719, 1.6617) -> (47.6719, 1)
  line L186 (47.6719, 1) -> (45.6512, 1)
  spline S189 degree 2 poles (45.6512, 1) (45.49, 1) (45.3572, 1.1186) (45.3572, 1.2158) knots 0 0 0 1 2 2 2
  spline S190 degree 2 poles (45.3572, 1.2158) (45.3572, 1.3131) (45.49, 1.4293) (45.6512, 1.4293) knots 0 0 0 1 2 2 2
  line L187 (45.6512, 1.4293) -> (45.7177, 1.4293)
  line L188 (45.7177, 1.4293) -> (45.7177, 3.1107)
  line L189 (45.7177, 3.1107) -> (45.6512, 3.1107)
  spline S191 degree 2 poles (45.6512, 3.1107) (45.49, 3.1107) (45.3572, 3.2293) (45.3572, 3.3266) knots 0 0 0 1 2 2 2
  spline S192 degree 2 poles (45.3572, 3.3266) (45.3572, 3.4214) (45.49, 3.54) (45.6512, 3.54) knots 0 0 0 1 2 2 2
  line L190 (45.6512, 3.54) -> (47.577, 3.5376)
  line L191 (47.577, 3.5376) -> (47.577, 2.8878)
  spline S193 degree 2 poles (47.577, 2.8878) (47.577, 2.7265) (47.4608, 2.5937) (47.3636, 2.5937) knots 0 0 0 1 2 2 2
  spline S194 degree 2 poles (47.3636, 2.5937) (47.2663, 2.5937) (47.1477, 2.7265) (47.1477, 2.8878) knots 0 0 0 1 2 2 2
  line L192 (47.1477, 2.8878) -> (47.1477, 3.1107)
  line L193 (47.1477, 3.1107) -> (46.1469, 3.1107)
  line L194 (46.1469, 3.1107) -> (46.1469, 2.4894)
  line L195 (46.1469, 2.4894) -> (46.524, 2.4894)
  spline S195 degree 2 poles (46.524, 2.4894) (46.524, 2.6506) (46.5619, 2.6933) knots 0 0 0 1 1 1
  spline S196 degree 2 poles (46.5619, 2.6933) (46.6426, 2.7835) (46.7398, 2.7835) knots 0 0 0 1 1 1
  spline S197 degree 2 poles (46.7398, 2.7835) (46.8371, 2.7835) (46.9533, 2.6506) (46.9533, 2.4894) knots 0 0 0 1 2 2 2
  line L196 (46.9533, 2.4894) -> (46.9533, 2.0601)
  spline S198 degree 2 poles (46.9533, 2.0601) (46.9533, 1.8988) (46.9153, 1.8538) knots 0 0 0 1 1 1
  spline S199 degree 2 poles (46.9153, 1.8538) (46.8371, 1.766) (46.7398, 1.766) knots 0 0 0 1 1 1
  spline S200 degree 2 poles (46.7398, 1.766) (46.6426, 1.766) (46.5619, 1.8562) knots 0 0 0 1 1 1
  spline S201 degree 2 poles (46.5619, 1.8562) (46.524, 1.8988) (46.524, 2.0601) knots 0 0 0 1 1 1
  line L197 (46.524, 2.0601) -> (46.1469, 2.0601)
  spline S202 degree 2 poles (48.5328, 1.1091) (48.4758, 1.0427) (48.4071, 1.0047) (48.3573, 1.0047) knots 0 0 0 1 2 2 2
  spline S203 degree 2 poles (48.3573, 1.0047) (48.2577, 1.0047) (48.1391, 1.1376) (48.1391, 1.2893) knots 0 0 0 1 2 2 2
  line L198 (48.1391, 1.2893) -> (48.1391, 1.5787)
  spline S204 degree 2 poles (48.1391, 1.5787) (48.1391, 1.7328) (48.2577, 1.8656) (48.3573, 1.8656) knots 0 0 0 1 2 2 2
  spline S205 degree 2 poles (48.3573, 1.8656) (48.4331, 1.8656) (48.5351, 1.785) (48.5897, 1.6) (48.6181, 1.5668) knots 0 0 0 1 2 3 3 3
  spline S206 degree 2 poles (48.6181, 1.5668) (48.6798, 1.5004) (48.9881, 1.3676) (49.1707, 1.3676) knots 0 0 0 1 2 2 2
  spline S207 degree 2 poles (49.1707, 1.3676) (49.4577, 1.3676) (49.6427, 1.5004) knots 0 0 0 1 1 1
  spline S208 degree 2 poles (49.6427, 1.5004) (49.7589, 1.5834) (49.7589, 1.702) knots 0 0 0 1 1 1
  spline S209 degree 2 poles (49.7589, 1.702) (49.7589, 1.7826) (49.6474, 1.9226) (49.5193, 1.9676) knots 0 0 0 1 2 2 2
  spline S210 degree 2 poles (49.5193, 1.9676) (49.4363, 1.9985) (49.147, 2.053) knots 0 0 0 1 1 1
  spline S211 degree 2 poles (49.147, 2.053) (48.796, 2.1194) (48.4355, 2.302) (48.2244, 2.6364) (48.2244, 2.8309) knots 0 0 0 1 2 3 3 3
  spline S212 degree 2 poles (48.2244, 2.8309) (48.2244, 3.1392) (48.7391, 3.6017) (49.1517, 3.6017) knots 0 0 0 1 2 2 2
  spline S213 degree 2 poles (49.1517, 3.6017) (49.3178, 3.6017) (49.6, 3.5281) (49.7162, 3.4523) knots 0 0 0 1 2 2 2
  spline S214 degree 2 poles (49.7162, 3.4523) (49.7992, 3.5353) (49.8846, 3.5353) knots 0 0 0 1 1 1
  spline S215 degree 2 poles (49.8846, 3.5353) (49.9794, 3.5353) (50.098, 3.4024) (50.098, 3.2507) knots 0 0 0 1 2 2 2
  line L199 (50.098, 3.2507) -> (50.098, 2.9281)
  spline S216 degree 2 poles (50.098, 2.9281) (50.098, 2.774) (49.9794, 2.6412) (49.8846, 2.6412) knots 0 0 0 1 2 2 2
  spline S217 degree 2 poles (49.8846, 2.6412) (49.8063, 2.6412) (49.747, 2.6886) knots 0 0 0 1 1 1
  spline S218 degree 2 poles (49.747, 2.6886) (49.6996, 2.7242) (49.6545, 2.9376) (49.619, 2.985) knots 0 0 0 1 2 2 2
  spline S219 degree 2 poles (49.619, 2.985) (49.5573, 3.0633) (49.3154, 3.1724) (49.1565, 3.1724) knots 0 0 0 1 2 2 2
  spline S220 degree 2 poles (49.1565, 3.1724) (48.9241, 3.1724) (48.6537, 2.9566) (48.6537, 2.8404) knots 0 0 0 1 2 2 2
  spline S221 degree 2 poles (48.6537, 2.8404) (48.6537, 2.7597) (48.7652, 2.6127) (48.8695, 2.57) knots 0 0 0 1 2 2 2
  spline S222 degree 2 poles (48.8695, 2.57) (48.9407, 2.5416) (49.5976, 2.4111) (49.9534, 2.257) (50.1881, 1.9249) (50.1881, 1.6973) knots 0 0 0 1 2 3 4 4 4
  spline S223 degree 2 poles (50.1881, 1.6973) (50.1881, 1.3795) (49.9652, 1.1897) knots 0 0 0 1 1 1
  spline S224 degree 2 poles (49.9652, 1.1897) (49.6664, 0.9383) (49.2063, 0.9383) knots 0 0 0 1 1 1
  spline S225 degree 2 poles (49.2063, 0.9383) (49.0284, 0.9383) (48.6917, 1.0237) (48.5328, 1.1091) knots 0 0 0 1 2 2 2
  spline S226 degree 2 poles (51.106, 1.1091) (51.049, 1.0427) (50.9803, 1.0047) (50.9305, 1.0047) knots 0 0 0 1 2 2 2
  spline S227 degree 2 poles (50.9305, 1.0047) (50.8309, 1.0047) (50.7123, 1.1376) (50.7123, 1.2893) knots 0 0 0 1 2 2 2
  line L200 (50.7123, 1.2893) -> (50.7123, 1.5787)
  spline S228 degree 2 poles (50.7123, 1.5787) (50.7123, 1.7328) (50.8309, 1.8656) (50.9305, 1.8656) knots 0 0 0 1 2 2 2
  spline S229 degree 2 poles (50.9305, 1.8656) (51.0064, 1.8656) (51.1083, 1.785) (51.1629, 1.6) (51.1913, 1.5668) knots 0 0 0 1 2 3 3 3
  spline S230 degree 2 poles (51.1913, 1.5668) (51.253, 1.5004) (51.5613, 1.3676) (51.7439, 1.3676) knots 0 0 0 1 2 2 2
  spline S231 degree 2 poles (51.7439, 1.3676) (52.0309, 1.3676) (52.2159, 1.5004) knots 0 0 0 1 1 1
  spline S232 degree 2 poles (52.2159, 1.5004) (52.3321, 1.5834) (52.3321, 1.702) knots 0 0 0 1 1 1
  spline S233 degree 2 poles (52.3321, 1.702) (52.3321, 1.7826) (52.2206, 1.9226) (52.0926, 1.9676) knots 0 0 0 1 2 2 2
  spline S234 degree 2 poles (52.0926, 1.9676) (52.0095, 1.9985) (51.7202, 2.053) knots 0 0 0 1 1 1
  spline S235 degree 2 poles (51.7202, 2.053) (51.3692, 2.1194) (51.0087, 2.302) (50.7977, 2.6364) (50.7977, 2.8309) knots 0 0 0 1 2 3 3 3
  spline S236 degree 2 poles (50.7977, 2.8309) (50.7977, 3.1392) (51.3123, 3.6017) (51.725, 3.6017) knots 0 0 0 1 2 2 2
  spline S237 degree 2 poles (51.725, 3.6017) (51.891, 3.6017) (52.1732, 3.5281) (52.2894, 3.4523) knots 0 0 0 1 2 2 2
  spline S238 degree 2 poles (52.2894, 3.4523) (52.3724, 3.5353) (52.4578, 3.5353) knots 0 0 0 1 1 1
  spline S239 degree 2 poles (52.4578, 3.5353) (52.5526, 3.5353) (52.6712, 3.4024) (52.6712, 3.2507) knots 0 0 0 1 2 2 2
  line L201 (52.6712, 3.2507) -> (52.6712, 2.9281)
  spline S240 degree 2 poles (52.6712, 2.9281) (52.6712, 2.774) (52.5526, 2.6412) (52.4578, 2.6412) knots 0 0 0 1 2 2 2
  spline S241 degree 2 poles (52.4578, 2.6412) (52.3795, 2.6412) (52.3202, 2.6886) knots 0 0 0 1 1 1
  spline S242 degree 2 poles (52.3202, 2.6886) (52.2728, 2.7242) (52.2277, 2.9376) (52.1922, 2.985) knots 0 0 0 1 2 2 2
  spline S243 degree 2 poles (52.1922, 2.985) (52.1305, 3.0633) (51.8886, 3.1724) (51.7297, 3.1724) knots 0 0 0 1 2 2 2
  spline S244 degree 2 poles (51.7297, 3.1724) (51.4973, 3.1724) (51.2269, 2.9566) (51.2269, 2.8404) knots 0 0 0 1 2 2 2
  spline S245 degree 2 poles (51.2269, 2.8404) (51.2269, 2.7597) (51.3384, 2.6127) (51.4427, 2.57) knots 0 0 0 1 2 2 2
  spline S246 degree 2 poles (51.4427, 2.57) (51.5139, 2.5416) (52.1708, 2.4111) (52.5266, 2.257) (52.7613, 1.9249) (52.7613, 1.6973) knots 0 0 0 1 2 3 4 4 4
  spline S247 degree 2 poles (52.7613, 1.6973) (52.7613, 1.3795) (52.5384, 1.1897) knots 0 0 0 1 1 1
  spline S248 degree 2 poles (52.5384, 1.1897) (52.2396, 0.9383) (51.7795, 0.9383) knots 0 0 0 1 1 1
  spline S249 degree 2 poles (51.7795, 0.9383) (51.6016, 0.9383) (51.2649, 1.0237) (51.106, 1.1091) knots 0 0 0 1 2 2 2
  line L202 (55.1899, 3.661) -> (53.812, 0.6964)
  spline S250 degree 2 poles (53.812, 0.6964) (53.7598, 0.585) (53.7171, 0.5518) knots 0 0 0 1 1 1
  spline S251 degree 2 poles (53.7171, 0.5518) (53.6649, 0.5067) (53.5867, 0.5067) knots 0 0 0 1 1 1
  spline S252 degree 2 poles (53.5867, 0.5067) (53.4989, 0.5067) (53.3732, 0.6324) (53.3732, 0.713) knots 0 0 0 1 2 2 2
  spline S253 degree 2 poles (53.3732, 0.713) (53.3732, 0.7676) (53.423, 0.8767) knots 0 0 0 1 1 1
  line L203 (53.423, 0.8767) -> (54.8033, 3.8388)
  spline S254 degree 2 poles (54.8033, 3.8388) (54.8555, 3.9503) (54.8958, 3.9835) knots 0 0 0 1 1 1
  spline S255 degree 2 poles (54.8958, 3.9835) (54.9503, 4.0286) (55.0262, 4.0286) knots 0 0 0 1 1 1
  spline S256 degree 2 poles (55.0262, 4.0286) (55.114, 4.0286) (55.2397, 3.9052) (55.2397, 3.8246) knots 0 0 0 1 2 2 2
  spline S257 degree 2 poles (55.2397, 3.8246) (55.2397, 3.77) (55.1899, 3.661) knots 0 0 0 1 1 1
  line L204 (55.9203, 1.4293) -> (55.9203, 3.1107)
  spline S258 degree 2 poles (55.9203, 3.1107) (55.7591, 3.1107) (55.6263, 3.2293) (55.6263, 3.3266) knots 0 0 0 1 2 2 2
  spline S259 degree 2 poles (55.6263, 3.3266) (55.6263, 3.4214) (55.7591, 3.54) (55.9203, 3.54) knots 0 0 0 1 2 2 2
  line L205 (55.9203, 3.54) -> (56.8263, 3.5376)
  spline S260 degree 2 poles (56.8263, 3.5376) (57.0374, 3.5376) (57.4429, 3.3835) (57.5639, 3.2625) knots 0 0 0 1 2 2 2
  spline S261 degree 2 poles (57.5639, 3.2625) (57.6587, 3.1724) (57.8579, 2.8593) (57.9599, 2.5487) (57.9599, 2.3257) knots 0 0 0 1 2 3 3 3
  line L206 (57.9599, 2.3257) -> (57.9599, 2.1194)
  spline S262 degree 2 poles (57.9599, 2.1194) (57.9599, 1.849) (57.7749, 1.4269) (57.4714, 1.1613) (57.3386, 1.0996) knots 0 0 0 1 2 3 3 3
  spline S263 degree 2 poles (57.3386, 1.0996) (57.1275, 1) (56.7907, 1) knots 0 0 0 1 1 1
  line L207 (56.7907, 1) -> (55.9203, 1)
  spline S264 degree 2 poles (55.9203, 1) (55.7591, 1) (55.6263, 1.1186) (55.6263, 1.2158) knots 0 0 0 1 2 2 2
  spline S265 degree 2 poles (55.6263, 1.2158) (55.6263, 1.3131) (55.7591, 1.4293) (55.9203, 1.4293) knots 0 0 0 1 2 2 2
  line L208 (56.3496, 1.4293) -> (56.805, 1.4293)
  spline S266 degree 2 poles (56.805, 1.4293) (57.0611, 1.4293) (57.1892, 1.5028) knots 0 0 0 1 1 1
  spline S267 degree 2 poles (57.1892, 1.5028) (57.3599, 1.6) (57.5307, 1.8965) (57.5307, 2.1336) knots 0 0 0 1 2 2 2
  line L209 (57.5307, 2.1336) -> (57.5307, 2.3376)
  spline S268 degree 2 poles (57.5307, 2.3376) (57.5307, 2.5416) (57.4524, 2.6933) knots 0 0 0 1 1 1
  spline S269 degree 2 poles (57.4524, 2.6933) (57.3315, 2.9329) (57.0279, 3.1107) (56.8002, 3.1107) knots 0 0 0 1 2 2 2
  line L210 (56.8002, 3.1107) -> (56.3496, 3.1107)
  line L211 (56.3496, 3.1107) -> (56.3496, 1.4293)
  line L212 (59.0129, 2.0601) -> (59.0129, 1.4293)
  line L213 (59.0129, 1.4293) -> (60.1086, 1.4293)
  line L214 (60.1086, 1.4293) -> (60.1086, 1.6617)
  spline S270 degree 2 poles (60.1086, 1.6617) (60.1086, 1.823) (60.2272, 1.9558) (60.3244, 1.9558) knots 0 0 0 1 2 2 2
  spline S271 degree 2 poles (60.3244, 1.9558) (60.4217, 1.9558) (60.5379, 1.823) (60.5379, 1.6617) knots 0 0 0 1 2 2 2
  line L215 (60.5379, 1.6617) -> (60.5379, 1)
  line L216 (60.5379, 1) -> (58.5173, 1)
  spline S272 degree 2 poles (58.5173, 1) (58.356, 1) (58.2232, 1.1186) (58.2232, 1.2158) knots 0 0 0 1 2 2 2
  spline S273 degree 2 poles (58.2232, 1.2158) (58.2232, 1.3131) (58.356, 1.4293) (58.5173, 1.4293) knots 0 0 0 1 2 2 2
  line L217 (58.5173, 1.4293) -> (58.5837, 1.4293)
  line L218 (58.5837, 1.4293) -> (58.5837, 3.1107)
  line L219 (58.5837, 3.1107) -> (58.5173, 3.1107)
  spline S274 degree 2 poles (58.5173, 3.1107) (58.356, 3.1107) (58.2232, 3.2293) (58.2232, 3.3266) knots 0 0 0 1 2 2 2
  spline S275 degree 2 poles (58.2232, 3.3266) (58.2232, 3.4214) (58.356, 3.54) (58.5173, 3.54) knots 0 0 0 1 2 2 2
  line L220 (58.5173, 3.54) -> (60.443, 3.5376)
  line L221 (60.443, 3.5376) -> (60.443, 2.8878)
  spline S276 degree 2 poles (60.443, 2.8878) (60.443, 2.7265) (60.3268, 2.5937) (60.2296, 2.5937) knots 0 0 0 1 2 2 2
  spline S277 degree 2 poles (60.2296, 2.5937) (60.1323, 2.5937) (60.0137, 2.7265) (60.0137, 2.8878) knots 0 0 0 1 2 2 2
  line L222 (60.0137, 2.8878) -> (60.0137, 3.1107)
  line L223 (60.0137, 3.1107) -> (59.0129, 3.1107)
  line L224 (59.0129, 3.1107) -> (59.0129, 2.4894)
  line L225 (59.0129, 2.4894) -> (59.39, 2.4894)
  spline S278 degree 2 poles (59.39, 2.4894) (59.39, 2.6506) (59.428, 2.6933) knots 0 0 0 1 1 1
  spline S279 degree 2 poles (59.428, 2.6933) (59.5086, 2.7835) (59.6058, 2.7835) knots 0 0 0 1 1 1
  spline S280 degree 2 poles (59.6058, 2.7835) (59.7031, 2.7835) (59.8193, 2.6506) (59.8193, 2.4894) knots 0 0 0 1 2 2 2
  line L226 (59.8193, 2.4894) -> (59.8193, 2.0601)
  spline S281 degree 2 poles (59.8193, 2.0601) (59.8193, 1.8988) (59.7813, 1.8538) knots 0 0 0 1 1 1
  spline S282 degree 2 poles (59.7813, 1.8538) (59.7031, 1.766) (59.6058, 1.766) knots 0 0 0 1 1 1
  spline S283 degree 2 poles (59.6058, 1.766) (59.5086, 1.766) (59.428, 1.8562) knots 0 0 0 1 1 1
  spline S284 degree 2 poles (59.428, 1.8562) (59.39, 1.8988) (59.39, 2.0601) knots 0 0 0 1 1 1
  line L227 (59.39, 2.0601) -> (59.0129, 2.0601)
  line L228 (61.4889, 2.7265) -> (61.4889, 1.4293)
  line L229 (61.4889, 1.4293) -> (61.643, 1.4293)
  spline S285 degree 2 poles (61.643, 1.4293) (61.8043, 1.4293) (61.9371, 1.3107) (61.9371, 1.2134) knots 0 0 0 1 2 2 2
  spline S286 degree 2 poles (61.9371, 1.2134) (61.9371, 1.1162) (61.8043, 1) (61.643, 1) knots 0 0 0 1 2 2 2
  line L230 (61.643, 1) -> (61.0596, 1)
  spline S287 degree 2 poles (61.0596, 1) (60.8984, 1) (60.7656, 1.1186) (60.7656, 1.2158) knots 0 0 0 1 2 2 2
  spline S288 degree 2 poles (60.7656, 1.2158) (60.7656, 1.3131) (60.8984, 1.4293) (61.0596, 1.4293) knots 0 0 0 1 2 2 2
  line L231 (61.0596, 1.4293) -> (61.0596, 3.1107)
  line L232 (61.0596, 3.1107) -> (60.9932, 3.1107)
  spline S289 degree 2 poles (60.9932, 3.1107) (60.832, 3.1107) (60.6991, 3.2293) (60.6991, 3.3266) knots 0 0 0 1 2 2 2
  spline S290 degree 2 poles (60.6991, 3.3266) (60.6991, 3.4214) (60.832, 3.54) (60.9932, 3.54) knots 0 0 0 1 2 2 2
  line L233 (60.9932, 3.54) -> (61.4865, 3.5376)
  line L234 (61.4865, 3.5376) -> (62.5893, 1.8158)
  line L235 (62.5893, 1.8158) -> (62.5893, 3.1107)
  line L236 (62.5893, 3.1107) -> (62.4352, 3.1107)
  spline S291 degree 2 poles (62.4352, 3.1107) (62.2739, 3.1107) (62.1411, 3.2293) (62.1411, 3.3266) knots 0 0 0 1 2 2 2
  spline S292 degree 2 poles (62.1411, 3.3266) (62.1411, 3.4214) (62.2739, 3.54) (62.4352, 3.54) knots 0 0 0 1 2 2 2
  line L237 (62.4352, 3.54) -> (63.0186, 3.5376)
  spline S293 degree 2 poles (63.0186, 3.5376) (63.1799, 3.5376) (63.3127, 3.4214) (63.3127, 3.3242) knots 0 0 0 1 2 2 2
  spline S294 degree 2 poles (63.3127, 3.3242) (63.3127, 3.2269) (63.1799, 3.1084) (63.0186, 3.1084) knots 0 0 0 1 2 2 2
  line L238 (63.0186, 3.1084) -> (63.0186, 1)
  line L239 (63.0186, 1) -> (62.5964, 1)
  line L240 (62.5964, 1) -> (61.4889, 2.7265)
  spline S295 degree 2 poles (64.0123, 1.1091) (63.9554, 1.0427) (63.8866, 1.0047) (63.8368, 1.0047) knots 0 0 0 1 2 2 2
  spline S296 degree 2 poles (63.8368, 1.0047) (63.7372, 1.0047) (63.6186, 1.1376) (63.6186, 1.2893) knots 0 0 0 1 2 2 2
  line L241 (63.6186, 1.2893) -> (63.6186, 1.5787)
  spline S297 degree 2 poles (63.6186, 1.5787) (63.6186, 1.7328) (63.7372, 1.8656) (63.8368, 1.8656) knots 0 0 0 1 2 2 2